Autodesk Inventor part; units mm, degrees
(part 5 of 6)
  arc A594 (139.7365, 123.5324) -> (139.7669, 123.0449) centre (147.3204, 123.76) ccw projected
  arc A595 (140.0993, 123.6997) -> (139.7365, 123.5324) centre (148.5, 105) ccw projected
  arc A596 (140.4503, 123.36) -> (140.0993, 123.6997) centre (135.0009, 118.0806) ccw projected
  arc A597 (140.7158, 123.0684) -> (140.4503, 123.36) centre (135.8481, 118.9014) ccw projected
  arc A598 (140.9107, 122.8267) -> (140.7158, 123.0684) centre (136.7109, 119.64) ccw projected
  arc A599 (141.2611, 122.9719) -> (140.9107, 122.8267) centre (148.5, 105) ccw projected
  arc A600 (141.228, 123.2805) -> (141.2611, 122.9719) centre (146.4841, 123.6882) ccw projected
  arc A601 (141.2096, 123.6745) -> (141.228, 123.2805) centre (147.6165, 123.776) ccw projected
  arc A602 (141.2175, 124.1629) -> (141.2096, 123.6745) centre (148.7959, 123.7947) ccw projected
  arc A603 (141.5923, 124.3011) -> (141.2175, 124.1629) centre (148.5, 105) ccw projected
  arc A604 (141.9156, 123.9349) -> (141.5923, 124.3011) centre (136.0688, 119.0994) ccw projected
  arc A605 (142.1575, 123.6234) -> (141.9156, 123.9349) centre (136.9778, 119.8512) ccw projected
  arc A606 (142.3327, 123.3672) -> (142.1575, 123.6234) centre (137.8959, 120.5199) ccw projected
  arc A607 (142.6934, 123.4844) -> (142.3327, 123.3672) centre (148.5, 105) ccw projected
  arc A608 (142.6846, 123.7947) -> (142.6934, 123.4844) centre (147.9566, 123.7888) ccw projected
  arc A609 (142.6972, 124.1889) -> (142.6846, 123.7947) centre (149.0924, 123.7875) ccw projected
  arc A610 (142.7435, 124.6752) -> (142.6972, 124.1889) centre (150.2696, 123.7136) ccw projected
  arc A611 (143.128, 124.7836) -> (142.7435, 124.6752) centre (148.5, 105) ccw projected
  arc A612 (143.4215, 124.3932) -> (143.128, 124.7836) centre (137.2133, 120.0313) ccw projected
  arc A613 (143.6382, 124.0636) -> (143.4215, 124.3932) centre (138.1785, 120.7095) ccw projected
  arc A614 (143.7928, 123.7945) -> (143.6382, 124.0636) centre (139.1463, 121.304) ccw projected
  arc A615 (144.1616, 123.883) -> (143.7928, 123.7945) centre (148.5, 105) ccw projected
  arc A616 (144.1772, 124.193) -> (144.1616, 123.883) centre (149.4324, 123.7735) ccw projected
  arc A617 (144.2207, 124.585) -> (144.1772, 124.193) centre (150.5646, 123.6831) ccw projected
  arc A618 (144.3049, 125.0662) -> (144.2207, 124.585) centre (151.7324, 123.517) ccw projected
  arc A619 (144.6967, 125.1441) -> (144.3049, 125.0662) centre (148.5, 105) ccw projected
  arc A620 (144.9587, 124.7318) -> (144.6967, 125.1441) centre (138.4274, 120.8705) ccw projected
  arc A621 (145.1489, 124.3863) -> (144.9587, 124.7318) centre (139.4429, 121.4708) ccw projected
  arc A622 (145.2819, 124.1059) -> (145.1489, 124.3863) centre (140.4543, 121.9876) ccw projected
  arc A623 (145.6565, 124.1652) -> (145.2819, 124.1059) centre (148.5, 105) ccw projected
  arc A624 (145.6964, 124.473) -> (145.6565, 124.1652) centre (150.9025, 123.6425) ccw projected
  arc A625 (145.7705, 124.8604) -> (145.6964, 124.473) centre (152.0241, 123.4635) ccw projected
  arc A626 (145.8922, 125.3335) -> (145.7705, 124.8604) centre (153.1753, 123.2064) ccw projected
  arc A627 (146.2889, 125.3804) -> (145.8922, 125.3335) centre (148.5, 105) ccw projected
  arc A628 (146.5178, 124.9489) -> (146.2889, 125.3804) centre (139.7037, 121.6119) ccw projected
  arc A629 (146.6803, 124.5895) -> (146.5178, 124.9489) centre (140.7631, 122.1307) ccw projected
  arc A630 (146.7909, 124.2995) -> (146.6803, 124.5895) centre (141.8119, 122.5665) ccw projected
  arc A631 (147.169, 124.3292) -> (146.7909, 124.2995) centre (148.5, 105) ccw projected
  arc A632 (147.2329, 124.633) -> (147.169, 124.3292) centre (152.3577, 123.3965) ccw projected
  arc A633 (147.3371, 125.0133) -> (147.2329, 124.633) centre (153.4618, 123.1301) ccw projected
  arc A634 (147.4956, 125.4754) -> (147.3371, 125.0133) centre (154.5894, 122.7834) ccw projected
  arc A635 (147.8948, 125.4911) -> (147.4956, 125.4754) centre (148.5, 105) ccw projected
  arc A636 (148.0891, 125.0429) -> (147.8948, 125.4911) centre (141.0342, 122.2508) ccw projected
  arc A637 (148.2229, 124.6719) -> (148.0891, 125.0429) centre (142.131, 122.6849) ccw projected
  arc A638 (148.3104, 124.3741) -> (148.2229, 124.6719) centre (143.2108, 123.0371) ccw projected
  arc A639 (148.6896, 124.3741) -> (148.3104, 124.3741) centre (148.5, 105) ccw projected
  arc A640 (148.7771, 124.6719) -> (148.6896, 124.3741) centre (153.7892, 123.0371) ccw projected
  circle A641 centre (148.5, 105) radius 6
  circle A642 centre (148.5, 105) radius 18.25
  point P0 (0, 0)
  dimension "d15" = 12
  dimension "d16" = 36.5
  constraints: 2 centre point, 2 coincident
  measures "d15" diameter of A641
  measures "d16" diameter of A642
extrude "押し出し4" cut sketch "スケッチ4" against normal blind 0.75 contours A642
fillet "フィレット1" radius 0.5 20 edges at (145.1332, 103.3479, -2.5) (144.8051, 104.3575, -2.5) (144.8051, 105.6424, -2.5) (145.1331, 106.652, -2.5) (145.8883, 107.6915, -2.5) (146.7471, 108.3155, -2.5) (147.9691, 108.7126, -2.5) (149.0314, 108.7125, -2.5) (150.2528, 108.3155, -2.5) (151.1126, 107.6906, -2.5) (151.8668, 106.6521, -2.5) (152.1951, 105.6411, -2.5) (152.1949, 104.3576, -2.5) (151.8663, 103.3467, -2.5) (151.1117, 102.3085, -2.5) (150.2516, 101.6838, -2.5) (149.0308, 101.2874, -2.5) (147.9686, 101.2875, -2.5) (146.7478, 101.6841, -2.5) (145.8884, 102.3084, -2.5)
sketch "スケッチ5" plane through (148.5, 105, 0.75) normal (0, 0, -1) x (-1, 0, 0)
  circle A0 centre (0, 0) radius 6 projected
  circle A1 centre (0, 0) radius 18.25 projected
  circle A2 centre (0, 0) radius 2 projected
  arc A3 (-0.2771, 19.6719) -> (-0.4109, 20.0429) centre (-6.369, 17.6849) ccw projected
  arc A4 (-0.1896, 19.3741) -> (-0.2771, 19.6719) centre (-5.2892, 18.0371) ccw projected
  arc A5 (0.1896, 19.3741) -> (-0.1896, 19.3741) centre (0, 0) ccw projected
  arc A6 (0.2771, 19.6719) -> (0.1896, 19.3741) centre (5.2892, 18.0371) ccw projected
  arc A7 (0.4109, 20.0429) -> (0.2771, 19.6719) centre (6.369, 17.6849) ccw projected
  arc A8 (0.6052, 20.4911) -> (0.4109, 20.0429) centre (7.4658, 17.2508) ccw projected
  arc A9 (1.0044, 20.4754) -> (0.6052, 20.4911) centre (0, 0) ccw projected
  arc A10 (1.1629, 20.0133) -> (1.0044, 20.4754) centre (-6.0894, 17.7834) ccw projected
  arc A11 (1.2671, 19.633) -> (1.1629, 20.0133) centre (-4.9618, 18.1301) ccw projected
  arc A12 (1.331, 19.3292) -> (1.2671, 19.633) centre (-3.8577, 18.3965) ccw projected
  arc A13 (1.7091, 19.2995) -> (1.331, 19.3292) centre (0, 0) ccw projected
  arc A14 (1.8197, 19.5895) -> (1.7091, 19.2995) centre (6.6881, 17.5665) ccw projected
  arc A15 (1.9822, 19.9489) -> (1.8197, 19.5895) centre (7.7369, 17.1307) ccw projected
  arc A16 (2.2111, 20.3804) -> (1.9822, 19.9489) centre (8.7963, 16.6119) ccw projected
  arc A17 (2.6078, 20.3335) -> (2.2111, 20.3804) centre (0, 0) ccw projected
  arc A18 (2.7295, 19.8604) -> (2.6078, 20.3335) centre (-4.6753, 18.2064) ccw projected
  arc A19 (2.8036, 19.473) -> (2.7295, 19.8604) centre (-3.5241, 18.4635) ccw projected
  arc A20 (2.8435, 19.1652) -> (2.8036, 19.473) centre (-2.4025, 18.6425) ccw projected
  arc A21 (3.2181, 19.1059) -> (2.8435, 19.1652) centre (0, 0) ccw projected
  arc A22 (3.3511, 19.3863) -> (3.2181, 19.1059) centre (8.0457, 16.9876) ccw projected
  arc A23 (3.5413, 19.7318) -> (3.3511, 19.3863) centre (9.0571, 16.4708) ccw projected
  arc A24 (3.8033, 20.1441) -> (3.5413, 19.7318) centre (10.0726, 15.8705) ccw projected
  arc A25 (4.1951, 20.0662) -> (3.8033, 20.1441) centre (0, 0) ccw projected
  arc A26 (4.2793, 19.585) -> (4.1951, 20.0662) centre (-3.2324, 18.517) ccw projected
  arc A27 (4.3228, 19.193) -> (4.2793, 19.585) centre (-2.0646, 18.6831) ccw projected
  arc A28 (4.3384, 18.883) -> (4.3228, 19.193) centre (-0.9324, 18.7735) ccw projected
  arc A29 (4.7072, 18.7945) -> (4.3384, 18.883) centre (0, 0) ccw projected
  arc A30 (4.8618, 19.0636) -> (4.7072, 18.7945) centre (9.3537, 16.304) ccw projected
  arc A31 (5.0785, 19.3932) -> (4.8618, 19.0636) centre (10.3215, 15.7095) ccw projected
  arc A32 (5.372, 19.7836) -> (5.0785, 19.3932) centre (11.2867, 15.0313) ccw projected
  arc A33 (5.7565, 19.6752) -> (5.372, 19.7836) centre (0, 0) ccw projected
  arc A34 (5.8028, 19.1889) -> (5.7565, 19.6752) centre (-1.7696, 18.7136) ccw projected
  arc A35 (5.8154, 18.7947) -> (5.8028, 19.1889) centre (-0.5924, 18.7875) ccw projected
  arc A36 (5.8066, 18.4844) -> (5.8154, 18.7947) centre (0.5434, 18.7888) ccw projected
  arc A37 (6.1673, 18.3672) -> (5.8066, 18.4844) centre (0, 0) ccw projected
  arc A38 (6.3425, 18.6234) -> (6.1673, 18.3672) centre (10.6041, 15.5199) ccw projected
  arc A39 (6.5844, 18.9349) -> (6.3425, 18.6234) centre (11.5222, 14.8512) ccw projected
  arc A40 (6.9077, 19.3011) -> (6.5844, 18.9349) centre (12.4312, 14.0994) ccw projected
  arc A41 (7.2825, 19.1629) -> (6.9077, 19.3011) centre (0, 0) ccw projected
  arc A42 (7.2904, 18.6745) -> (7.2825, 19.1629) centre (-0.2959, 18.7947) ccw projected
  arc A43 (7.272, 18.2805) -> (7.2904, 18.6745) centre (0.8835, 18.776) ccw projected
  arc A44 (7.2389, 17.9719) -> (7.272, 18.2805) centre (2.0159, 18.6882) ccw projected
  arc A45 (7.5893, 17.8267) -> (7.2389, 17.9719) centre (0, 0) ccw projected
  arc A46 (7.7842, 18.0684) -> (7.5893, 17.8267) centre (11.7891, 14.64) ccw projected
  arc A47 (8.0497, 18.36) -> (7.7842, 18.0684) centre (12.6519, 13.9014) ccw projected
  arc A48 (8.4007, 18.6997) -> (8.0497, 18.36) centre (13.4991, 13.0806) ccw projected
  arc A49 (8.7635, 18.5324) -> (8.4007, 18.6997) centre (0, 0) ccw projected
  arc A50 (8.7331, 18.0449) -> (8.7635, 18.5324) centre (1.1796, 18.76) ccw projected
  arc A51 (8.6839, 17.6536) -> (8.7331, 18.0449) centre (2.3539, 18.6488) ccw projected
  arc A52 (8.6267, 17.3485) -> (8.6839, 17.6536) centre (3.476, 18.4724) ccw projected
  arc A53 (8.9646, 17.1763) -> (8.6267, 17.3485) centre (0, 0) ccw projected
  arc A54 (9.1778, 17.4019) -> (8.9646, 17.1763) centre (12.9014, 13.6699) ccw projected
  arc A55 (9.4654, 17.6718) -> (9.1778, 17.4019) centre (13.7036, 12.8659) ccw projected
  arc A56 (9.842, 17.9829) -> (9.4654, 17.6718) centre (14.4838, 11.9812) ccw projected
  arc A57 (10.1905, 17.7877) -> (9.842, 17.9829) centre (0, 0) ccw projected
  arc A58 (10.122, 17.3041) -> (10.1905, 17.7877) centre (2.6478, 18.6096) ccw projected
  arc A59 (10.0422, 16.9178) -> (10.122, 17.3041) centre (3.8099, 18.4067) ccw projected
  arc A60 (9.9612, 16.6182) -> (10.0422, 16.9178) centre (4.9146, 18.1428) ccw projected
  arc A61 (10.2846, 16.42) -> (9.9612, 16.6182) centre (0, 0) ccw projected
  arc A62 (10.5148, 16.6282) -> (10.2846, 16.42) centre (13.9341, 12.6156) ccw projected
  arc A63 (10.8227, 16.8747) -> (10.5148, 16.6282) centre (14.6708, 11.7511) ccw projected
  arc A64 (11.2226, 17.1553) -> (10.8227, 16.8747) centre (15.3792, 10.8078) ccw projected
  arc A65 (11.5547, 16.9334) -> (11.2226, 17.1553) centre (0, 0) ccw projected
  arc A66 (11.4485, 16.4566) -> (11.5547, 16.9334) centre (4.0998, 18.3445) ccw projected
  arc A67 (11.3386, 16.0778) -> (11.4485, 16.4566) centre (5.2423, 18.051) ccw projected
  arc A68 (11.2344, 15.7854) -> (11.3386, 16.0778) centre (6.3229, 17.7012) ccw projected
  arc A69 (11.5412, 15.5625) -> (11.2344, 15.7854) centre (0, 0) ccw projected
  arc A70 (11.7871, 15.752) -> (11.5412, 15.5625) centre (14.881, 11.4834) ccw projected
  arc A71 (12.1134, 15.9735) -> (11.7871, 15.752) centre (15.5476, 10.5638) ccw projected
  arc A72 (12.534, 16.2219) -> (12.1134, 15.9735) centre (16.1798, 9.5679) ccw projected
  arc A73 (12.8477, 15.9746) -> (12.534, 16.2219) centre (0, 0) ccw projected
  arc A74 (12.7043, 15.5076) -> (12.8477, 15.9746) centre (5.5264, 17.9663) ccw projected
  arc A75 (12.5651, 15.1386) -> (12.7043, 15.5076) centre (6.6424, 17.5841) ccw projected
  arc A76 (12.4383, 14.8553) -> (12.5651, 15.1386) centre (7.6922, 17.1506) ccw projected
  arc A77 (12.7266, 14.609) -> (12.4383, 14.8553) centre (0, 0) ccw projected
  arc A78 (12.9866, 14.7786) -> (12.7266, 14.609) centre (15.7361, 10.2805) ccw projected
  arc A79 (13.3293, 14.9739) -> (12.9866, 14.7786) centre (16.3285, 9.3114) ccw projected
  arc A80 (13.7681, 15.1885) -> (13.3293, 14.9739) centre (16.8806, 8.2689) ccw projected
  arc A81 (14.0614, 14.9173) -> (13.7681, 15.1885) centre (0, 0) ccw projected
  arc A82 (13.8819, 14.463) -> (14.0614, 14.9173) centre (6.919, 17.4773) ccw projected
  arc A83 (13.7141, 14.1061) -> (13.8819, 14.463) centre (8.0015, 17.0087) ccw projected
  arc A84 (13.5655, 13.8336) -> (13.7141, 14.1061) centre (9.0141, 16.4942) ccw projected
  arc A85 (13.8336, 13.5655) -> (13.5655, 13.8336) centre (0, 0) ccw projected
  arc A86 (14.1061, 13.7141) -> (13.8336, 13.5655) centre (16.4942, 9.0141) ccw projected
  arc A87 (14.463, 13.8819) -> (14.1061, 13.7141) centre (17.0087, 8.0015) ccw projected
  arc A88 (14.9173, 14.0614) -> (14.463, 13.8819) centre (17.4773, 6.919) ccw projected
  arc A89 (15.1885, 13.7681) -> (14.9173, 14.0614) centre (0, 0) ccw projected
  arc A90 (14.9739, 13.3293) -> (15.1885, 13.7681) centre (8.2689, 16.8806) ccw projected
  arc A91 (14.7786, 12.9866) -> (14.9739, 13.3293) centre (9.3114, 16.3285) ccw projected
  arc A92 (14.609, 12.7266) -> (14.7786, 12.9866) centre (10.2805, 15.7361) ccw projected
  arc A93 (14.8553, 12.4383) -> (14.609, 12.7266) centre (0, 0) ccw projected
  arc A94 (15.1386, 12.5651) -> (14.8553, 12.4383) centre (17.1506, 7.6922) ccw projected
  arc A95 (15.5076, 12.7043) -> (15.1386, 12.5651) centre (17.5841, 6.6424) ccw projected
  arc A96 (15.9746, 12.8477) -> (15.5076, 12.7043) centre (17.9663, 5.5264) ccw projected
  arc A97 (16.2219, 12.534) -> (15.9746, 12.8477) centre (0, 0) ccw projected
  arc A98 (15.9735, 12.1134) -> (16.2219, 12.534) centre (9.5679, 16.1798) ccw projected
  arc A99 (15.752, 11.7871) -> (15.9735, 12.1134) centre (10.5638, 15.5476) ccw projected
  arc A100 (15.5625, 11.5412) -> (15.752, 11.7871) centre (11.4834, 14.881) ccw projected
  arc A101 (15.7854, 11.2344) -> (15.5625, 11.5412) centre (0, 0) ccw projected
  arc A102 (16.0778, 11.3386) -> (15.7854, 11.2344) centre (17.7012, 6.3229) ccw projected
  arc A103 (16.4566, 11.4485) -> (16.0778, 11.3386) centre (18.051, 5.2423) ccw projected
  arc A104 (16.9334, 11.5547) -> (16.4566, 11.4485) centre (18.3445, 4.0998) ccw projected
  arc A105 (17.1553, 11.2226) -> (16.9334, 11.5547) centre (0, 0) ccw projected
  arc A106 (16.8747, 10.8227) -> (17.1553, 11.2226) centre (10.8078, 15.3792) ccw projected
  arc A107 (16.6282, 10.5148) -> (16.8747, 10.8227) centre (11.7511, 14.6708) ccw projected
  arc A108 (16.42, 10.2846) -> (16.6282, 10.5148) centre (12.6156, 13.9341) ccw projected
  arc A109 (16.6182, 9.9612) -> (16.42, 10.2846) centre (0, 0) ccw projected
  arc A110 (16.9178, 10.0422) -> (16.6182, 9.9612) centre (18.1428, 4.9146) ccw projected
  arc A111 (17.3041, 10.122) -> (16.9178, 10.0422) centre (18.4067, 3.8099) ccw projected
  arc A112 (17.7877, 10.1905) -> (17.3041, 10.122) centre (18.6096, 2.6478) ccw projected
  arc A113 (17.9829, 9.842) -> (17.7877, 10.1905) centre (0, 0) ccw projected
  arc A114 (17.6718, 9.4654) -> (17.9829, 9.842) centre (11.9812, 14.4838) ccw projected
  arc A115 (17.4019, 9.1778) -> (17.6718, 9.4654) centre (12.8659, 13.7036) ccw projected
  arc A116 (17.1763, 8.9646) -> (17.4019, 9.1778) centre (13.6699, 12.9014) ccw projected
  arc A117 (17.3485, 8.6267) -> (17.1763, 8.9646) centre (0, 0) ccw projected
  arc A118 (17.6536, 8.6839) -> (17.3485, 8.6267) centre (18.4724, 3.476) ccw projected
  arc A119 (18.0449, 8.7331) -> (17.6536, 8.6839) centre (18.6488, 2.3539) ccw projected
  arc A120 (18.5324, 8.7635) -> (18.0449, 8.7331) centre (18.76, 1.1796) ccw projected
  arc A121 (18.6997, 8.4007) -> (18.5324, 8.7635) centre (0, 0) ccw projected
  arc A122 (18.36, 8.0497) -> (18.6997, 8.4007) centre (13.0806, 13.4991) ccw projected
  arc A123 (18.0684, 7.7842) -> (18.36, 8.0497) centre (13.9014, 12.6519) ccw projected
  arc A124 (17.8267, 7.5893) -> (18.0684, 7.7842) centre (14.64, 11.7891) ccw projected
  arc A125 (17.9719, 7.2389) -> (17.8267, 7.5893) centre (0, 0) ccw projected
  arc A126 (18.2805, 7.272) -> (17.9719, 7.2389) centre (18.6882, 2.0159) ccw projected
  arc A127 (18.6745, 7.2904) -> (18.2805, 7.272) centre (18.776, 0.8835) ccw projected
  arc A128 (19.1629, 7.2825) -> (18.6745, 7.2904) centre (18.7947, -0.2959) ccw projected
  arc A129 (19.3011, 6.9077) -> (19.1629, 7.2825) centre (0, 0) ccw projected
  arc A130 (18.9349, 6.5844) -> (19.3011, 6.9077) centre (14.0994, 12.4312) ccw projected
  arc A131 (18.6234, 6.3425) -> (18.9349, 6.5844) centre (14.8512, 11.5222) ccw projected
  arc A132 (18.3672, 6.1673) -> (18.6234, 6.3425) centre (15.5199, 10.6041) ccw projected
  arc A133 (18.4844, 5.8066) -> (18.3672, 6.1673) centre (0, 0) ccw projected
  arc A134 (18.7947, 5.8154) -> (18.4844, 5.8066) centre (18.7888, 0.5434) ccw projected
  arc A135 (19.1889, 5.8028) -> (18.7947, 5.8154) centre (18.7875, -0.5924) ccw projected
  arc A136 (19.6752, 5.7565) -> (19.1889, 5.8028) centre (18.7136, -1.7696) ccw projected
  arc A137 (19.7836, 5.372) -> (19.6752, 5.7565) centre (0, 0) ccw projected
  arc A138 (19.3932, 5.0785) -> (19.7836, 5.372) centre (15.0313, 11.2867) ccw projected
  arc A139 (19.0636, 4.8618) -> (19.3932, 5.0785) centre (15.7095, 10.3215) ccw projected
  arc A140 (18.7945, 4.7072) -> (19.0636, 4.8618) centre (16.304, 9.3537) ccw projected
  arc A141 (18.883, 4.3384) -> (18.7945, 4.7072) centre (0, 0) ccw projected
  arc A142 (19.193, 4.3228) -> (18.883, 4.3384) centre (18.7735, -0.9324) ccw projected
  arc A143 (19.585, 4.2793) -> (19.193, 4.3228) centre (18.6831, -2.0646) ccw projected
  arc A144 (20.0662, 4.1951) -> (19.585, 4.2793) centre (18.517, -3.2324) ccw projected
  arc A145 (20.1441, 3.8033) -> (20.0662, 4.1951) centre (0, 0) ccw projected
  arc A146 (19.7318, 3.5413) -> (20.1441, 3.8033) centre (15.8705, 10.0726) ccw projected
  arc A147 (19.3863, 3.3511) -> (19.7318, 3.5413) centre (16.4708, 9.0571) ccw projected
  arc A148 (19.1059, 3.2181) -> (19.3863, 3.3511) centre (16.9876, 8.0457) ccw projected
  arc A149 (19.1652, 2.8435) -> (19.1059, 3.2181) centre (0, 0) ccw projected
  arc A150 (19.473, 2.8036) -> (19.1652, 2.8435) centre (18.6425, -2.4025) ccw projected
  arc A151 (19.8604, 2.7295) -> (19.473, 2.8036) centre (18.4635, -3.5241) ccw projected
  arc A152 (20.3335, 2.6078) -> (19.8604, 2.7295) centre (18.2064, -4.6753) ccw projected
  arc A153 (20.3804, 2.2111) -> (20.3335, 2.6078) centre (0, 0) ccw projected
  arc A154 (19.9489, 1.9822) -> (20.3804, 2.2111) centre (16.6119, 8.7963) ccw projected
  arc A155 (19.5895, 1.8197) -> (19.9489, 1.9822) centre (17.1307, 7.7369) ccw projected
  arc A156 (19.2995, 1.7091) -> (19.5895, 1.8197) centre (17.5665, 6.6881) ccw projected
  arc A157 (19.3292, 1.331) -> (19.2995, 1.7091) centre (0, 0) ccw projected
  arc A158 (19.633, 1.2671) -> (19.3292, 1.331) centre (18.3965, -3.8577) ccw projected
  arc A159 (20.0133, 1.1629) -> (19.633, 1.2671) centre (18.1301, -4.9618) ccw projected
  arc A160 (20.4754, 1.0044) -> (20.0133, 1.1629) centre (17.7834, -6.0894) ccw projected
  arc A161 (20.4911, 0.6052) -> (20.4754, 1.0044) centre (0, 0) ccw projected
  arc A162 (20.0429, 0.4109) -> (20.4911, 0.6052) centre (17.2508, 7.4658) ccw projected
  arc A163 (19.6719, 0.2771) -> (20.0429, 0.4109) centre (17.6849, 6.369) ccw projected
  arc A164 (19.3741, 0.1896) -> (19.6719, 0.2771) centre (18.0371, 5.2892) ccw projected
  arc A165 (19.3741, -0.1896) -> (19.3741, 0.1896) centre (0, 0) ccw projected
  arc A166 (19.6719, -0.2771) -> (19.3741, -0.1896) centre (18.0371, -5.2892) ccw projected
  arc A167 (20.0429, -0.4109) -> (19.6719, -0.2771) centre (17.6849, -6.369) ccw projected
  arc A168 (20.4911, -0.6052) -> (20.0429, -0.4109) centre (17.2508, -7.4658) ccw projected
  arc A169 (20.4754, -1.0044) -> (20.4911, -0.6052) centre (0, 0) ccw projected
  arc A170 (20.0133, -1.1629) -> (20.4754, -1.0044) centre (17.7834, 6.0894) ccw projected
  arc A171 (19.633, -1.2671) -> (20.0133, -1.1629) centre (18.1301, 4.9618) ccw projected
  arc A172 (19.3292, -1.331) -> (19.633, -1.2671) centre (18.3965, 3.8577) ccw projected
  arc A173 (19.2995, -1.7091) -> (19.3292, -1.331) centre (0, 0) ccw projected
  arc A174 (19.5895, -1.8197) -> (19.2995, -1.7091) centre (17.5665, -6.6881) ccw projected
  arc A175 (19.9489, -1.9822) -> (19.5895, -1.8197) centre (17.1307, -7.7369) ccw projected
  arc A176 (20.3804, -2.2111) -> (19.9489, -1.9822) centre (16.6119, -8.7963) ccw projected
  arc A177 (20.3335, -2.6078) -> (20.3804, -2.2111) centre (0, 0) ccw projected
  arc A178 (19.8604, -2.7295) -> (20.3335, -2.6078) centre (18.2064, 4.6753) ccw projected
  arc A179 (19.473, -2.8036) -> (19.8604, -2.7295) centre (18.4635, 3.5241) ccw projected
  arc A180 (19.1652, -2.8435) -> (19.473, -2.8036) centre (18.6425, 2.4025) ccw projected
  arc A181 (19.1059, -3.2181) -> (19.1652, -2.8435) centre (0, 0) ccw projected
  arc A182 (19.3863, -3.3511) -> (19.1059, -3.2181) centre (16.9876, -8.0457) ccw projected
  arc A183 (19.7318, -3.5413) -> (19.3863, -3.3511) centre (16.4708, -9.0571) ccw projected
  arc A184 (20.1441, -3.8033) -> (19.7318, -3.5413) centre (15.8705, -10.0726) ccw projected
  arc A185 (20.0662, -4.1951) -> (20.1441, -3.8033) centre (0, 0) ccw projected
  arc A186 (19.585, -4.2793) -> (20.0662, -4.1951) centre (18.517, 3.2324) ccw projected
  arc A187 (19.193, -4.3228) -> (19.585, -4.2793) centre (18.6831, 2.0646) ccw projected
  arc A188 (18.883, -4.3384) -> (19.193, -4.3228) centre (18.7735, 0.9324) ccw projected
  arc A189 (18.7945, -4.7072) -> (18.883, -4.3384) centre (0, 0) ccw projected
  arc A190 (19.0636, -4.8618) -> (18.7945, -4.7072) centre (16.304, -9.3537) ccw projected
  arc A191 (19.3932, -5.0785) -> (19.0636, -4.8618) centre (15.7095, -10.3215) ccw projected
  arc A192 (19.7836, -5.372) -> (19.3932, -5.0785) centre (15.0313, -11.2867) ccw projected
  arc A193 (19.6752, -5.7565) -> (19.7836, -5.372) centre (0, 0) ccw projected
  arc A194 (19.1889, -5.8028) -> (19.6752, -5.7565) centre (18.7136, 1.7696) ccw projected
  arc A195 (18.7947, -5.8154) -> (19.1889, -5.8028) centre (18.7875, 0.5924) ccw projected
  arc A196 (18.4844, -5.8066) -> (18.7947, -5.8154) centre (18.7888, -0.5434) ccw projected
  arc A197 (18.3672, -6.1673) -> (18.4844, -5.8066) centre (0, 0) ccw projected
  arc A198 (18.6234, -6.3425) -> (18.3672, -6.1673) centre (15.5199, -10.6041) ccw projected
  arc A199 (18.9349, -6.5844) -> (18.6234, -6.3425) centre (14.8512, -11.5222) ccw projected
  arc A200 (19.3011, -6.9077) -> (18.9349, -6.5844) centre (14.0994, -12.4312) ccw projected
  arc A201 (19.1629, -7.2825) -> (19.3011, -6.9077) centre (0, 0) ccw projected
  arc A202 (18.6745, -7.2904) -> (19.1629, -7.2825) centre (18.7947, 0.2959) ccw projected
  arc A203 (18.2805, -7.272) -> (18.6745, -7.2904) centre (18.776, -0.8835) ccw projected
  arc A204 (17.9719, -7.2389) -> (18.2805, -7.272) centre (18.6882, -2.0159) ccw projected
  arc A205 (17.8267, -7.5893) -> (17.9719, -7.2389) centre (0, 0) ccw projected
  arc A206 (18.0684, -7.7842) -> (17.8267, -7.5893) centre (14.64, -11.7891) ccw projected
  arc A207 (18.36, -8.0497) -> (18.0684, -7.7842) centre (13.9014, -12.6519) ccw projected
  arc A208 (18.6997, -8.4007) -> (18.36, -8.0497) centre (13.0806, -13.4991) ccw projected
  arc A209 (18.5324, -8.7635) -> (18.6997, -8.4007) centre (0, 0) ccw projected
  arc A210 (18.0449, -8.7331) -> (18.5324, -8.7635) centre (18.76, -1.1796) ccw projected
  arc A211 (17.6536, -8.6839) -> (18.0449, -8.7331) centre (18.6488, -2.3539) ccw projected
  arc A212 (17.3485, -8.6267) -> (17.6536, -8.6839) centre (18.4724, -3.476) ccw projected
  arc A213 (17.1763, -8.9646) -> (17.3485, -8.6267) centre (0, 0) ccw projected
  arc A214 (17.4019, -9.1778) -> (17.1763, -8.9646) centre (13.6699, -12.9014) ccw projected
  arc A215 (17.6718, -9.4654) -> (17.4019, -9.1778) centre (12.8659, -13.7036) ccw projected
  arc A216 (17.9829, -9.842) -> (17.6718, -9.4654) centre (11.9812, -14.4838) ccw projected
  arc A217 (17.7877, -10.1905) -> (17.9829, -9.842) centre (0, 0) ccw projected
  arc A218 (17.3041, -10.122) -> (17.7877, -10.1905) centre (18.6096, -2.6478) ccw projected
  arc A219 (16.9178, -10.0422) -> (17.3041, -10.122) centre (18.4067, -3.8099) ccw projected
  arc A220 (16.6182, -9.9612) -> (16.9178, -10.0422) centre (18.1428, -4.9146) ccw projected
  arc A221 (16.42, -10.2846) -> (16.6182, -9.9612) centre (0, 0) ccw projected
  arc A222 (16.6282, -10.5148) -> (16.42, -10.2846) centre (12.6156, -13.9341) ccw projected
  arc A223 (16.8747, -10.8227) -> (16.6282, -10.5148) centre (11.7511, -14.6708) ccw projected
  arc A224 (17.1553, -11.2226) -> (16.8747, -10.8227) centre (10.8078, -15.3792) ccw projected
  arc A225 (16.9334, -11.5547) -> (17.1553, -11.2226) centre (0, 0) ccw projected
  arc A226 (16.4566, -11.4485) -> (16.9334, -11.5547) centre (18.3445, -4.0998) ccw projected
  arc A227 (16.0778, -11.3386) -> (16.4566, -11.4485) centre (18.051, -5.2423) ccw projected
  arc A228 (15.7854, -11.2344) -> (16.0778, -11.3386) centre (17.7012, -6.3229) ccw projected
  arc A229 (15.5625, -11.5412) -> (15.7854, -11.2344) centre (0, 0) ccw projected
  arc A230 (15.752, -11.7871) -> (15.5625, -11.5412) centre (11.4834, -14.881) ccw projected
  arc A231 (15.9735, -12.1134) -> (15.752, -11.7871) centre (10.5638, -15.5476) ccw projected
  arc A232 (16.2219, -12.534) -> (15.9735, -12.1134) centre (9.5679, -16.1798) ccw projected
  arc A233 (15.9746, -12.8477) -> (16.2219, -12.534) centre (0, 0) ccw projected
  arc A234 (15.5076, -12.7043) -> (15.9746, -12.8477) centre (17.9663, -5.5264) ccw projected
  arc A235 (15.1386, -12.5651) -> (15.5076, -12.7043) centre (17.5841, -6.6424) ccw projected
  arc A236 (14.8553, -12.4383) -> (15.1386, -12.5651) centre (17.1506, -7.6922) ccw projected
  arc A237 (14.609, -12.7266) -> (14.8553, -12.4383) centre (0, 0) ccw projected
  arc A238 (14.7786, -12.9866) -> (14.609, -12.7266) centre (10.2805, -15.7361) ccw projected
  arc A239 (14.9739, -13.3293) -> (14.7786, -12.9866) centre (9.3114, -16.3285) ccw projected
  arc A240 (15.1885, -13.7681) -> (14.9739, -13.3293) centre (8.2689, -16.8806) ccw projected
  arc A241 (14.9173, -14.0614) -> (15.1885, -13.7681) centre (0, 0) ccw projected
  arc A242 (14.463, -13.8819) -> (14.9173, -14.0614) centre (17.4773, -6.919) ccw projected
  arc A243 (14.1061, -13.7141) -> (14.463, -13.8819) centre (17.0087, -8.0015) ccw projected
  arc A244 (13.8336, -13.5655) -> (14.1061, -13.7141) centre (16.4942, -9.0141) ccw projected
  arc A245 (13.5655, -13.8336) -> (13.8336, -13.5655) centre (0, 0) ccw projected
  arc A246 (13.7141, -14.1061) -> (13.5655, -13.8336) centre (9.0141, -16.4942) ccw projected
  arc A247 (13.8819, -14.463) -> (13.7141, -14.1061) centre (8.0015, -17.0087) ccw projected
  arc A248 (14.0614, -14.9173) -> (13.8819, -14.463) centre (6.919, -17.4773) ccw projected
  arc A249 (13.7681, -15.1885) -> (14.0614, -14.9173) centre (0, 0) ccw projected
  arc A250 (13.3293, -14.9739) -> (13.7681, -15.1885) centre (16.8806, -8.2689) ccw projected
  arc A251 (12.9866, -14.7786) -> (13.3293, -14.9739) centre (16.3285, -9.3114) ccw projected
  arc A252 (12.7266, -14.609) -> (12.9866, -14.7786) centre (15.7361, -10.2805) ccw projected
  arc A253 (12.4383, -14.8553) -> (12.7266, -14.609) centre (0, 0) ccw projected
  arc A254 (12.5651, -15.1386) -> (12.4383, -14.8553) centre (7.6922, -17.1506) ccw projected
  arc A255 (12.7043, -15.5076) -> (12.5651, -15.1386) centre (6.6424, -17.5841) ccw projected
  arc A256 (12.8477, -15.9746) -> (12.7043, -15.5076) centre (5.5264, -17.9663) ccw projected
  arc A257 (12.534, -16.2219) -> (12.8477, -15.9746) centre (0, 0) ccw projected
  arc A258 (12.1134, -15.9735) -> (12.534, -16.2219) centre (16.1798, -9.5679) ccw projected
  arc A259 (11.7871, -15.752) -> (12.1134, -15.9735) centre (15.5476, -10.5638) ccw projected
  arc A260 (11.5412, -15.5625) -> (11.7871, -15.752) centre (14.881, -11.4834) ccw projected
  arc A261 (11.2344, -15.7854) -> (11.5412, -15.5625) centre (0, 0) ccw projected
  arc A262 (11.3386, -16.0778) -> (11.2344, -15.7854) centre (6.3229, -17.7012) ccw projected
  arc A263 (11.4485, -16.4566) -> (11.3386, -16.0778) centre (5.2423, -18.051) ccw projected
  arc A264 (11.5547, -16.9334) -> (11.4485, -16.4566) centre (4.0998, -18.3445) ccw projected
  arc A265 (11.2226, -17.1553) -> (11.5547, -16.9334) centre (0, 0) ccw projected
  arc A266 (10.8227, -16.8747) -> (11.2226, -17.1553) centre (15.3792, -10.8078) ccw projected
  arc A267 (10.5148, -16.6282) -> (10.8227, -16.8747) centre (14.6708, -11.7511) ccw projected
  arc A268 (10.2846, -16.42) -> (10.5148, -16.6282) centre (13.9341, -12.6156) ccw projected
  arc A269 (9.9612, -16.6182) -> (10.2846, -16.42) centre (0, 0) ccw projected
  arc A270 (10.0422, -16.9178) -> (9.9612, -16.6182) centre (4.9146, -18.1428) ccw projected
  arc A271 (10.122, -17.3041) -> (10.0422, -16.9178) centre (3.8099, -18.4067) ccw projected
  arc A272 (10.1905, -17.7877) -> (10.122, -17.3041) centre (2.6478, -18.6096) ccw projected
  arc A273 (9.842, -17.9829) -> (10.1905, -17.7877) centre (0, 0) ccw projected
  arc A274 (9.4654, -17.6718) -> (9.842, -17.9829) centre (14.4838, -11.9812) ccw projected
  arc A275 (9.1778, -17.4019) -> (9.4654, -17.6718) centre (13.7036, -12.8659) ccw projected
  arc A276 (8.9646, -17.1763) -> (9.1778, -17.4019) centre (12.9014, -13.6699) ccw projected
  arc A277 (8.6267, -17.3485) -> (8.9646, -17.1763) centre (0, 0) ccw projected
  arc A278 (8.6839, -17.6536) -> (8.6267, -17.3485) centre (3.476, -18.4724) ccw projected
  arc A279 (8.7331, -18.0449) -> (8.6839, -17.6536) centre (2.3539, -18.6488) ccw projected
  arc A280 (8.7635, -18.5324) -> (8.7331, -18.0449) centre (1.1796, -18.76) ccw projected
  arc A281 (8.4007, -18.6997) -> (8.7635, -18.5324) centre (0, 0) ccw projected
  arc A282 (8.0497, -18.36) -> (8.4007, -18.6997) centre (13.4991, -13.0806) ccw projected
  arc A283 (7.7842, -18.0684) -> (8.0497, -18.36) centre (12.6519, -13.9014) ccw projected
  arc A284 (7.5893, -17.8267) -> (7.7842, -18.0684) centre (11.7891, -14.64) ccw projected
  arc A285 (7.2389, -17.9719) -> (7.5893, -17.8267) centre (0, 0) ccw projected
  arc A286 (7.272, -18.2805) -> (7.2389, -17.9719) centre (2.0159, -18.6882) ccw projected
  arc A287 (7.2904, -18.6745) -> (7.272, -18.2805) centre (0.8835, -18.776) ccw projected
  arc A288 (7.2825, -19.1629) -> (7.2904, -18.6745) centre (-0.2959, -18.7947) ccw projected
  arc A289 (6.9077, -19.3011) -> (7.2825, -19.1629) centre (0, 0) ccw projected
  arc A290 (6.5844, -18.9349) -> (6.9077, -19.3011) centre (12.4312, -14.0994) ccw projected
  arc A291 (6.3425, -18.6234) -> (6.5844, -18.9349) centre (11.5222, -14.8512) ccw projected
  arc A292 (6.1673, -18.3672) -> (6.3425, -18.6234) centre (10.6041, -15.5199) ccw projected
  arc A293 (5.8066, -18.4844) -> (6.1673, -18.3672) centre (0, 0) ccw projected
  arc A294 (5.8154, -18.7947) -> (5.8066, -18.4844) centre (0.5434, -18.7888) ccw projected
  arc A295 (5.8028, -19.1889) -> (5.8154, -18.7947) centre (-0.5924, -18.7875) ccw projected
  arc A296 (5.7565, -19.6752) -> (5.8028, -19.1889) centre (-1.7696, -18.7136) ccw projected
  arc A297 (5.372, -19.7836) -> (5.7565, -19.6752) centre (0, 0) ccw projected
  arc A298 (5.0785, -19.3932) -> (5.372, -19.7836) centre (11.2867, -15.0313) ccw projected
  arc A299 (4.8618, -19.0636) -> (5.0785, -19.3932) centre (10.3215, -15.7095) ccw projected
  arc A300 (4.7072, -18.7945) -> (4.8618, -19.0636) centre (9.3537, -16.304) ccw projected
  arc A301 (4.3384, -18.883) -> (4.7072, -18.7945) centre (0, 0) ccw projected
  arc A302 (4.3228, -19.193) -> (4.3384, -18.883) centre (-0.9324, -18.7735) ccw projected
  arc A303 (4.2793, -19.585) -> (4.3228, -19.193) centre (-2.0646, -18.6831) ccw projected
  arc A304 (4.1951, -20.0662) -> (4.2793, -19.585) centre (-3.2324, -18.517) ccw projected
  arc A305 (3.8033, -20.1441) -> (4.1951, -20.0662) centre (0, 0) ccw projected
  arc A306 (3.5413, -19.7318) -> (3.8033, -20.1441) centre (10.0726, -15.8705) ccw projected
  arc A307 (3.3511, -19.3863) -> (3.5413, -19.7318) centre (9.0571, -16.4708) ccw projected
  arc A308 (3.2181, -19.1059) -> (3.3511, -19.3863) centre (8.0457, -16.9876) ccw projected
  arc A309 (2.8435, -19.1652) -> (3.2181, -19.1059) centre (0, 0) ccw projected
  arc A310 (2.8036, -19.473) -> (2.8435, -19.1652) centre (-2.4025, -18.6425) ccw projected
  arc A311 (2.7295, -19.8604) -> (2.8036, -19.473) centre (-3.5241, -18.4635) ccw projected
  arc A312 (2.6078, -20.3335) -> (2.7295, -19.8604) centre (-4.6753, -18.2064) ccw projected
  arc A313 (2.2111, -20.3804) -> (2.6078, -20.3335) centre (0, 0) ccw projected
  arc A314 (1.9822, -19.9489) -> (2.2111, -20.3804) centre (8.7963, -16.6119) ccw projected
  arc A315 (1.8197, -19.5895) -> (1.9822, -19.9489) centre (7.7369, -17.1307) ccw projected
  arc A316 (1.7091, -19.2995) -> (1.8197, -19.5895) centre (6.6881, -17.5665) ccw projected
  arc A317 (1.331, -19.3292) -> (1.7091, -19.2995) centre (0, 0) ccw projected
  arc A318 (1.2671, -19.633) -> (1.331, -19.3292) centre (-3.8577, -18.3965) ccw projected
  arc A319 (1.1629, -20.0133) -> (1.2671, -19.633) centre (-4.9618, -18.1301) ccw projected
  arc A320 (1.0044, -20.4754) -> (1.1629, -20.0133) centre (-6.0894, -17.7834) ccw projected
  arc A321 (0.6052, -20.4911) -> (1.0044, -20.4754) centre (0, 0) ccw projected
  arc A322 (0.4109, -20.0429) -> (0.6052, -20.4911) centre (7.4658, -17.2508) ccw projected
  arc A323 (0.2771, -19.6719) -> (0.4109, -20.0429) centre (6.369, -17.6849) ccw projected
  arc A324 (0.1896, -19.3741) -> (0.2771, -19.6719) centre (5.2892, -18.0371) ccw projected
  arc A325 (-0.1896, -19.3741) -> (0.1896, -19.3741) centre (0, 0) ccw projected
  arc A326 (-0.2771, -19.6719) -> (-0.1896, -19.3741) centre (-5.2892, -18.0371) ccw projected
  arc A327 (-0.4109, -20.0429) -> (-0.2771, -19.6719) centre (-6.369, -17.6849) ccw projected
  arc A328 (-0.6052, -20.4911) -> (-0.4109, -20.0429) centre (-7.4658, -17.2508) ccw projected
  arc A329 (-1.0044, -20.4754) -> (-0.6052, -20.4911) centre (0, 0) ccw projected
  arc A330 (-1.1629, -20.0133) -> (-1.0044, -20.4754) centre (6.0894, -17.7834) ccw projected
  arc A331 (-1.2671, -19.633) -> (-1.1629, -20.0133) centre (4.9618, -18.1301) ccw projected
  arc A332 (-1.331, -19.3292) -> (-1.2671, -19.633) centre (3.8577, -18.3965) ccw projected
  arc A333 (-1.7091, -19.2995) -> (-1.331, -19.3292) centre (0, 0) ccw projected
  arc A334 (-1.8197, -19.5895) -> (-1.7091, -19.2995) centre (-6.6881, -17.5665) ccw projected
  arc A335 (-1.9822, -19.9489) -> (-1.8197, -19.5895) centre (-7.7369, -17.1307) ccw projected
  arc A336 (-2.2111, -20.3804) -> (-1.9822, -19.9489) centre (-8.7963, -16.6119) ccw projected
  arc A337 (-2.6078, -20.3335) -> (-2.2111, -20.3804) centre (0, 0) ccw projected
  arc A338 (-2.7295, -19.8604) -> (-2.6078, -20.3335) centre (4.6753, -18.2064) ccw projected
  arc A339 (-2.8036, -19.473) -> (-2.7295, -19.8604) centre (3.5241, -18.4635) ccw projected
  arc A340 (-2.8435, -19.1652) -> (-2.8036, -19.473) centre (2.4025, -18.6425) ccw projected
  arc A341 (-3.2181, -19.1059) -> (-2.8435, -19.1652) centre (0, 0) ccw projected
  arc A342 (-3.3511, -19.3863) -> (-3.2181, -19.1059) centre (-8.0457, -16.9876) ccw projected
  arc A343 (-3.5413, -19.7318) -> (-3.3511, -19.3863) centre (-9.0571, -16.4708) ccw projected
  arc A344 (-3.8033, -20.1441) -> (-3.5413, -19.7318) centre (-10.0726, -15.8705) ccw projected
  arc A345 (-4.1951, -20.0662) -> (-3.8033, -20.1441) centre (0, 0) ccw projected
  arc A346 (-4.2793, -19.585) -> (-4.1951, -20.0662) centre (3.2324, -18.517) ccw projected
  arc A347 (-4.3228, -19.193) -> (-4.2793, -19.585) centre (2.0646, -18.6831) ccw projected
  arc A348 (-4.3384, -18.883) -> (-4.3228, -19.193) centre (0.9324, -18.7735) ccw projected
  arc A349 (-4.7072, -18.7945) -> (-4.3384, -18.883) centre (0, 0) ccw projected
  arc A350 (-4.8618, -19.0636) -> (-4.7072, -18.7945) centre (-9.3537, -16.304) ccw projected
  arc A351 (-5.0785, -19.3932) -> (-4.8618, -19.0636) centre (-10.3215, -15.7095) ccw projected
  arc A352 (-5.372, -19.7836) -> (-5.0785, -19.3932) centre (-11.2867, -15.0313) ccw projected
  arc A353 (-5.7565, -19.6752) -> (-5.372, -19.7836) centre (0, 0) ccw projected
  arc A354 (-5.8028, -19.1889) -> (-5.7565, -19.6752) centre (1.7696, -18.7136) ccw projected
  arc A355 (-5.8154, -18.7947) -> (-5.8028, -19.1889) centre (0.5924, -18.7875) ccw projected
  arc A356 (-5.8066, -18.4844) -> (-5.8154, -18.7947) centre (-0.5434, -18.7888) ccw projected
  arc A357 (-6.1673, -18.3672) -> (-5.8066, -18.4844) centre (0, 0) ccw projected
  arc A358 (-6.3425, -18.6234) -> (-6.1673, -18.3672) centre (-10.6041, -15.5199) ccw projected
  arc A359 (-6.5844, -18.9349) -> (-6.3425, -18.6234) centre (-11.5222, -14.8512) ccw projected
  arc A360 (-6.9077, -19.3011) -> (-6.5844, -18.9349) centre (-12.4312, -14.0994) ccw projected
  arc A361 (-7.2825, -19.1629) -> (-6.9077, -19.3011) centre (0, 0) ccw projected
  arc A362 (-7.2904, -18.6745) -> (-7.2825, -19.1629) centre (0.2959, -18.7947) ccw projected
  arc A363 (-7.272, -18.2805) -> (-7.2904, -18.6745) centre (-0.8835, -18.776) ccw projected
  arc A364 (-7.2389, -17.9719) -> (-7.272, -18.2805) centre (-2.0159, -18.6882) ccw projected
  arc A365 (-7.5893, -17.8267) -> (-7.2389, -17.9719) centre (0, 0) ccw projected
  arc A366 (-7.7842, -18.0684) -> (-7.5893, -17.8267) centre (-11.7891, -14.64) ccw projected
  arc A367 (-8.0497, -18.36) -> (-7.7842, -18.0684) centre (-12.6519, -13.9014) ccw projected
  arc A368 (-8.4007, -18.6997) -> (-8.0497, -18.36) centre (-13.4991, -13.0806) ccw projected
  arc A369 (-8.7635, -18.5324) -> (-8.4007, -18.6997) centre (0, 0) ccw projected
  arc A370 (-8.7331, -18.0449) -> (-8.7635, -18.5324) centre (-1.1796, -18.76) ccw projected
  arc A371 (-8.6839, -17.6536) -> (-8.7331, -18.0449) centre (-2.3539, -18.6488) ccw projected
  arc A372 (-8.6267, -17.3485) -> (-8.6839, -17.6536) centre (-3.476, -18.4724) ccw projected
  arc A373 (-8.9646, -17.1763) -> (-8.6267, -17.3485) centre (0, 0) ccw projected
  arc A374 (-9.1778, -17.4019) -> (-8.9646, -17.1763) centre (-12.9014, -13.6699) ccw projected
  arc A375 (-9.4654, -17.6718) -> (-9.1778, -17.4019) centre (-13.7036, -12.8659) ccw projected
  arc A376 (-9.842, -17.9829) -> (-9.4654, -17.6718) centre (-14.4838, -11.9812) ccw projected
  arc A377 (-10.1905, -17.7877) -> (-9.842, -17.9829) centre (0, 0) ccw projected
  arc A378 (-10.122, -17.3041) -> (-10.1905, -17.7877) centre (-2.6478, -18.6096) ccw projected
  arc A379 (-10.0422, -16.9178) -> (-10.122, -17.3041) centre (-3.8099, -18.4067) ccw projected
  arc A380 (-9.9612, -16.6182) -> (-10.0422, -16.9178) centre (-4.9146, -18.1428) ccw projected
  arc A381 (-10.2846, -16.42) -> (-9.9612, -16.6182) centre (0, 0) ccw projected
  arc A382 (-10.5148, -16.6282) -> (-10.2846, -16.42) centre (-13.9341, -12.6156) ccw projected
  arc A383 (-10.8227, -16.8747) -> (-10.5148, -16.6282) centre (-14.6708, -11.7511) ccw projected
  arc A384 (-11.2226, -17.1553) -> (-10.8227, -16.8747) centre (-15.3792, -10.8078) ccw projected
  arc A385 (-11.5547, -16.9334) -> (-11.2226, -17.1553) centre (0, 0) ccw projected
  arc A386 (-11.4485, -16.4566) -> (-11.5547, -16.9334) centre (-4.0998, -18.3445) ccw projected
  arc A387 (-11.3386, -16.0778) -> (-11.4485, -16.4566) centre (-5.2423, -18.051) ccw projected
  arc A388 (-11.2344, -15.7854) -> (-11.3386, -16.0778) centre (-6.3229, -17.7012) ccw projected
  arc A389 (-11.5412, -15.5625) -> (-11.2344, -15.7854) centre (0, 0) ccw projected
  arc A390 (-11.7871, -15.752) -> (-11.5412, -15.5625) centre (-14.881, -11.4834) ccw projected
  arc A391 (-12.1134, -15.9735) -> (-11.7871, -15.752) centre (-15.5476, -10.5638) ccw projected
  arc A392 (-12.534, -16.2219) -> (-12.1134, -15.9735) centre (-16.1798, -9.5679) ccw projected
  arc A393 (-12.8477, -15.9746) -> (-12.534, -16.2219) centre (0, 0) ccw projected
  arc A394 (-12.7043, -15.5076) -> (-12.8477, -15.9746) centre (-5.5264, -17.9663) ccw projected
  arc A395 (-12.5651, -15.1386) -> (-12.7043, -15.5076) centre (-6.6424, -17.5841) ccw projected
  arc A396 (-12.4383, -14.8553) -> (-12.5651, -15.1386) centre (-7.6922, -17.1506) ccw projected
  arc A397 (-12.7266, -14.609) -> (-12.4383, -14.8553) centre (0, 0) ccw projected
  arc A398 (-12.9866, -14.7786) -> (-12.7266, -14.609) centre (-15.7361, -10.2805) ccw projected
  arc A399 (-13.3293, -14.9739) -> (-12.9866, -14.7786) centre (-16.3285, -9.3114) ccw projected
  arc A400 (-13.7681, -15.1885) -> (-13.3293, -14.9739) centre (-16.8806, -8.2689) ccw projected
  arc A401 (-14.0614, -14.9173) -> (-13.7681, -15.1885) centre (0, 0) ccw projected
  arc A402 (-13.8819, -14.463) -> (-14.0614, -14.9173) centre (-6.919, -17.4773) ccw projected
  arc A403 (-13.7141, -14.1061) -> (-13.8819, -14.463) centre (-8.0015, -17.0087) ccw projected
  arc A404 (-13.5655, -13.8336) -> (-13.7141, -14.1061) centre (-9.0141, -16.4942) ccw projected
  arc A405 (-13.8336, -13.5655) -> (-13.5655, -13.8336) centre (0, 0) ccw projected
  arc A406 (-14.1061, -13.7141) -> (-13.8336, -13.5655) centre (-16.4942, -9.0141) ccw projected
  arc A407 (-14.463, -13.8819) -> (-14.1061, -13.7141) centre (-17.0087, -8.0015) ccw projected
  arc A408 (-14.9173, -14.0614) -> (-14.463, -13.8819) centre (-17.4773, -6.919) ccw projected
  arc A409 (-15.1885, -13.7681) -> (-14.9173, -14.0614) centre (0, 0) ccw projected
  arc A410 (-14.9739, -13.3293) -> (-15.1885, -13.7681) centre (-8.2689, -16.8806) ccw projected
  arc A411 (-14.7786, -12.9866) -> (-14.9739, -13.3293) centre (-9.3114, -16.3285) ccw projected
  arc A412 (-14.609, -12.7266) -> (-14.7786, -12.9866) centre (-10.2805, -15.7361) ccw projected
  arc A413 (-14.8553, -12.4383) -> (-14.609, -12.7266) centre (0, 0) ccw projected
  arc A414 (-15.1386, -12.5651) -> (-14.8553, -12.4383) centre (-17.1506, -7.6922) ccw projected
  arc A415 (-15.5076, -12.7043) -> (-15.1386, -12.5651) centre (-17.5841, -6.6424) ccw projected
  arc A416 (-15.9746, -12.8477) -> (-15.5076, -12.7043) centre (-17.9663, -5.5264) ccw projected
  arc A417 (-16.2219, -12.534) -> (-15.9746, -12.8477) centre (0, 0) ccw projected
  arc A418 (-15.9735, -12.1134) -> (-16.2219, -12.534) centre (-9.5679, -16.1798) ccw projected
  arc A419 (-15.752, -11.7871) -> (-15.9735, -12.1134) centre (-10.5638, -15.5476) ccw projected
  arc A420 (-15.5625, -11.5412) -> (-15.752, -11.7871) centre (-11.4834, -14.881) ccw projected
  arc A421 (-15.7854, -11.2344) -> (-15.5625, -11.5412) centre (0, 0) ccw projected
  arc A422 (-16.0778, -11.3386) -> (-15.7854, -11.2344) centre (-17.7012, -6.3229) ccw projected
  arc A423 (-16.4566, -11.4485) -> (-16.0778, -11.3386) centre (-18.051, -5.2423) ccw projected
  arc A424 (-16.9334, -11.5547) -> (-16.4566, -11.4485) centre (-18.3445, -4.0998) ccw projected
  arc A425 (-17.1553, -11.2226) -> (-16.9334, -11.5547) centre (0, 0) ccw projected
  arc A426 (-16.8747, -10.8227) -> (-17.1553, -11.2226) centre (-10.8078, -15.3792) ccw projected
  arc A427 (-16.6282, -10.5148) -> (-16.8747, -10.8227) centre (-11.7511, -14.6708) ccw projected
  arc A428 (-16.42, -10.2846) -> (-16.6282, -10.5148) centre (-12.6156, -13.9341) ccw projected
  arc A429 (-16.6182, -9.9612) -> (-16.42, -10.2846) centre (0, 0) ccw projected
  arc A430 (-16.9178, -10.0422) -> (-16.6182, -9.9612) centre (-18.1428, -4.9146) ccw projected
  arc A431 (-17.3041, -10.122) -> (-16.9178, -10.0422) centre (-18.4067, -3.8099) ccw projected
  arc A432 (-17.7877, -10.1905) -> (-17.3041, -10.122) centre (-18.6096, -2.6478) ccw projected
  arc A433 (-17.9829, -9.842) -> (-17.7877, -10.1905) centre (0, 0) ccw projected
  arc A434 (-17.6718, -9.4654) -> (-17.9829, -9.842) centre (-11.9812, -14.4838) ccw projected
  arc A435 (-17.4019, -9.1778) -> (-17.6718, -9.4654) centre (-12.8659, -13.7036) ccw projected
  arc A436 (-17.1763, -8.9646) -> (-17.4019, -9.1778) centre (-13.6699, -12.9014) ccw projected
  arc A437 (-17.3485, -8.6267) -> (-17.1763, -8.9646) centre (0, 0) ccw projected
  arc A438 (-17.6536, -8.6839) -> (-17.3485, -8.6267) centre (-18.4724, -3.476) ccw projected
  arc A439 (-18.0449, -8.7331) -> (-17.6536, -8.6839) centre (-18.6488, -2.3539) ccw projected
  arc A440 (-18.5324, -8.7635) -> (-18.0449, -8.7331) centre (-18.76, -1.1796) ccw projected
  arc A441 (-18.6997, -8.4007) -> (-18.5324, -8.7635) centre (0, 0) ccw projected
  arc A442 (-18.36, -8.0497) -> (-18.6997, -8.4007) centre (-13.0806, -13.4991) ccw projected
  arc A443 (-18.0684, -7.7842) -> (-18.36, -8.0497) centre (-13.9014, -12.6519) ccw projected
  arc A444 (-17.8267, -7.5893) -> (-18.0684, -7.7842) centre (-14.64, -11.7891) ccw projected
  arc A445 (-17.9719, -7.2389) -> (-17.8267, -7.5893) centre (0, 0) ccw projected
  arc A446 (-18.2805, -7.272) -> (-17.9719, -7.2389) centre (-18.6882, -2.0159) ccw projected
  arc A447 (-18.6745, -7.2904) -> (-18.2805, -7.272) centre (-18.776, -0.8835) ccw projected
  arc A448 (-19.1629, -7.2825) -> (-18.6745, -7.2904) centre (-18.7947, 0.2959) ccw projected
  arc A449 (-19.3011, -6.9077) -> (-19.1629, -7.2825) centre (0, 0) ccw projected
  arc A450 (-18.9349, -6.5844) -> (-19.3011, -6.9077) centre (-14.0994, -12.4312) ccw projected
  arc A451 (-18.6234, -6.3425) -> (-18.9349, -6.5844) centre (-14.8512, -11.5222) ccw projected
  arc A452 (-18.3672, -6.1673) -> (-18.6234, -6.3425) centre (-15.5199, -10.6041) ccw projected
  arc A453 (-18.4844, -5.8066) -> (-18.3672, -6.1673) centre (0, 0) ccw projected
  arc A454 (-18.7947, -5.8154) -> (-18.4844, -5.8066) centre (-18.7888, -0.5434) ccw projected
  arc A455 (-19.1889, -5.8028) -> (-18.7947, -5.8154) centre (-18.7875, 0.5924) ccw projected
  arc A456 (-19.6752, -5.7565) -> (-19.1889, -5.8028) centre (-18.7136, 1.7696) ccw projected
  arc A457 (-19.7836, -5.372) -> (-19.6752, -5.7565) centre (0, 0) ccw projected
  arc A458 (-19.3932, -5.0785) -> (-19.7836, -5.372) centre (-15.0313, -11.2867) ccw projected
  arc A459 (-19.0636, -4.8618) -> (-19.3932, -5.0785) centre (-15.7095, -10.3215) ccw projected
  arc A460 (-18.7945, -4.7072) -> (-19.0636, -4.8618) centre (-16.304, -9.3537) ccw projected
  arc A461 (-18.883, -4.3384) -> (-18.7945, -4.7072) centre (0, 0) ccw projected
  arc A462 (-19.193, -4.3228) -> (-18.883, -4.3384) centre (-18.7735, 0.9324) ccw projected
  arc A463 (-19.585, -4.2793) -> (-19.193, -4.3228) centre (-18.6831, 2.0646) ccw projected
  arc A464 (-20.0662, -4.1951) -> (-19.585, -4.2793) centre (-18.517, 3.2324) ccw projected
  arc A465 (-20.1441, -3.8033) -> (-20.0662, -4.1951) centre (0, 0) ccw projected
  arc A466 (-19.7318, -3.5413) -> (-20.1441, -3.8033) centre (-15.8705, -10.0726) ccw projected
  arc A467 (-19.3863, -3.3511) -> (-19.7318, -3.5413) centre (-16.4708, -9.0571) ccw projected
  arc A468 (-19.1059, -3.2181) -> (-19.3863, -3.3511) centre (-16.9876, -8.0457) ccw projected
  arc A469 (-19.1652, -2.8435) -> (-19.1059, -3.2181) centre (0, 0) ccw projected
  arc A470 (-19.473, -2.8036) -> (-19.1652, -2.8435) centre (-18.6425, 2.4025) ccw projected
  arc A471 (-19.8604, -2.7295) -> (-19.473, -2.8036) centre (-18.4635, 3.5241) ccw projected
  arc A472 (-20.3335, -2.6078) -> (-19.8604, -2.7295) centre (-18.2064, 4.6753) ccw projected
  arc A473 (-20.3804, -2.2111) -> (-20.3335, -2.6078) centre (0, 0) ccw projected
  arc A474 (-19.9489, -1.9822) -> (-20.3804, -2.2111) centre (-16.6119, -8.7963) ccw projected
  arc A475 (-19.5895, -1.8197) -> (-19.9489, -1.9822) centre (-17.1307, -7.7369) ccw projected
  arc A476 (-19.2995, -1.7091) -> (-19.5895, -1.8197) centre (-17.5665, -6.6881) ccw projected
  arc A477 (-19.3292, -1.331) -> (-19.2995, -1.7091) centre (0, 0) ccw projected
  arc A478 (-19.633, -1.2671) -> (-19.3292, -1.331) centre (-18.3965, 3.8577) ccw projected
  arc A479 (-20.0133, -1.1629) -> (-19.633, -1.2671) centre (-18.1301, 4.9618) ccw projected
  arc A480 (-20.4754, -1.0044) -> (-20.0133, -1.1629) centre (-17.7834, 6.0894) ccw projected
  arc A481 (-20.4911, -0.6052) -> (-20.4754, -1.0044) centre (0, 0) ccw projected
  arc A482 (-20.0429, -0.4109) -> (-20.4911, -0.6052) centre (-17.2508, -7.4658) ccw projected
  arc A483 (-19.6719, -0.2771) -> (-20.0429, -0.4109) centre (-17.6849, -6.369) ccw projected
  arc A484 (-19.3741, -0.1896) -> (-19.6719, -0.2771) centre (-18.0371, -5.2892) ccw projected
  arc A485 (-19.3741, 0.1896) -> (-19.3741, -0.1896) centre (0, 0) ccw projected
  arc A486 (-19.6719, 0.2771) -> (-19.3741, 0.1896) centre (-18.0371, 5.2892) ccw projected
  arc A487 (-20.0429, 0.4109) -> (-19.6719, 0.2771) centre (-17.6849, 6.369) ccw projected
  arc A488 (-20.4911, 0.6052) -> (-20.0429, 0.4109) centre (-17.2508, 7.4658) ccw projected
  arc A489 (-20.4754, 1.0044) -> (-20.4911, 0.6052) centre (0, 0) ccw projected
  arc A490 (-20.0133, 1.1629) -> (-20.4754, 1.0044) centre (-17.7834, -6.0894) ccw projected
  arc A491 (-19.633, 1.2671) -> (-20.0133, 1.1629) centre (-18.1301, -4.9618) ccw projected
  arc A492 (-19.3292, 1.331) -> (-19.633, 1.2671) centre (-18.3965, -3.8577) ccw projected
  arc A493 (-19.2995, 1.7091) -> (-19.3292, 1.331) centre (0, 0) ccw projected
  arc A494 (-19.5895, 1.8197) -> (-19.2995, 1.7091) centre (-17.5665, 6.6881) ccw projected
  arc A495 (-19.9489, 1.9822) -> (-19.5895, 1.8197) centre (-17.1307, 7.7369) ccw projected
  arc A496 (-20.3804, 2.2111) -> (-19.9489, 1.9822) centre (-16.6119, 8.7963) ccw projected
  arc A497 (-20.3335, 2.6078) -> (-20.3804, 2.2111) centre (0, 0) ccw projected
  arc A498 (-19.8604, 2.7295) -> (-20.3335, 2.6078) centre (-18.2064, -4.6753) ccw projected
  arc A499 (-19.473, 2.8036) -> (-19.8604, 2.7295) centre (-18.4635, -3.5241) ccw projected
  arc A500 (-19.1652, 2.8435) -> (-19.473, 2.8036) centre (-18.6425, -2.4025) ccw projected
  arc A501 (-19.1059, 3.2181) -> (-19.1652, 2.8435) centre (0, 0) ccw projected
  arc A502 (-19.3863, 3.3511) -> (-19.1059, 3.2181) centre (-16.9876, 8.0457) ccw projected
  arc A503 (-19.7318, 3.5413) -> (-19.3863, 3.3511) centre (-16.4708, 9.0571) ccw projected
  arc A504 (-20.1441, 3.8033) -> (-19.7318, 3.5413) centre (-15.8705, 10.0726) ccw projected
  arc A505 (-20.0662, 4.1951) -> (-20.1441, 3.8033) centre (0, 0) ccw projected
  arc A506 (-19.585, 4.2793) -> (-20.0662, 4.1951) centre (-18.517, -3.2324) ccw projected
  arc A507 (-19.193, 4.3228) -> (-19.585, 4.2793) centre (-18.6831, -2.0646) ccw projected
  arc A508 (-18.883, 4.3384) -> (-19.193, 4.3228) centre (-18.7735, -0.9324) ccw projected
  arc A509 (-18.7945, 4.7072) -> (-18.883, 4.3384) centre (0, 0) ccw projected
  arc A510 (-19.0636, 4.8618) -> (-18.7945, 4.7072) centre (-16.304, 9.3537) ccw projected
  arc A511 (-19.3932, 5.0785) -> (-19.0636, 4.8618) centre (-15.7095, 10.3215) ccw projected
  arc A512 (-19.7836, 5.372) -> (-19.3932, 5.0785) centre (-15.0313, 11.2867) ccw projected
  arc A513 (-19.6752, 5.7565) -> (-19.7836, 5.372) centre (0, 0) ccw projected
  arc A514 (-19.1889, 5.8028) -> (-19.6752, 5.7565) centre (-18.7136, -1.7696) ccw projected
  arc A515 (-18.7947, 5.8154) -> (-19.1889, 5.8028) centre (-18.7875, -0.5924) ccw projected
  arc A516 (-18.4844, 5.8066) -> (-18.7947, 5.8154) centre (-18.7888, 0.5434) ccw projected
  arc A517 (-18.3672, 6.1673) -> (-18.4844, 5.8066) centre (0, 0) ccw projected
  arc A518 (-18.6234, 6.3425) -> (-18.3672, 6.1673) centre (-15.5199, 10.6041) ccw projected
  arc A519 (-18.9349, 6.5844) -> (-18.6234, 6.3425) centre (-14.8512, 11.5222) ccw projected
  arc A520 (-19.3011, 6.9077) -> (-18.9349, 6.5844) centre (-14.0994, 12.4312) ccw projected
  arc A521 (-19.1629, 7.2825) -> (-19.3011, 6.9077) centre (0, 0) ccw projected
  arc A522 (-18.6745, 7.2904) -> (-19.1629, 7.2825) centre (-18.7947, -0.2959) ccw projected
  arc A523 (-18.2805, 7.272) -> (-18.6745, 7.2904) centre (-18.776, 0.8835) ccw projected
  arc A524 (-17.9719, 7.2389) -> (-18.2805, 7.272) centre (-18.6882, 2.0159) ccw projected
  arc A525 (-17.8267, 7.5893) -> (-17.9719, 7.2389) centre (0, 0) ccw projected
  arc A526 (-18.0684, 7.7842) -> (-17.8267, 7.5893) centre (-14.64, 11.7891) ccw projected
  arc A527 (-18.36, 8.0497) -> (-18.0684, 7.7842) centre (-13.9014, 12.6519) ccw projected
  arc A528 (-18.6997, 8.4007) -> (-18.36, 8.0497) centre (-13.0806, 13.4991) ccw projected
  arc A529 (-18.5324, 8.7635) -> (-18.6997, 8.4007) centre (0, 0) ccw projected
  arc A530 (-18.0449, 8.7331) -> (-18.5324, 8.7635) centre (-18.76, 1.1796) ccw projected
  arc A531 (-17.6536, 8.6839) -> (-18.0449, 8.7331) centre (-18.6488, 2.3539) ccw projected
  arc A532 (-17.3485, 8.6267) -> (-17.6536, 8.6839) centre (-18.4724, 3.476) ccw projected
  arc A533 (-17.1763, 8.9646) -> (-17.3485, 8.6267) centre (0, 0) ccw projected
  arc A534 (-17.4019, 9.1778) -> (-17.1763, 8.9646) centre (-13.6699, 12.9014) ccw projected
  arc A535 (-17.6718, 9.4654) -> (-17.4019, 9.1778) centre (-12.8659, 13.7036) ccw projected
  arc A536 (-17.9829, 9.842) -> (-17.6718, 9.4654) centre (-11.9812, 14.4838) ccw projected
  arc A537 (-17.7877, 10.1905) -> (-17.9829, 9.842) centre (0, 0) ccw projected
  arc A538 (-17.3041, 10.122) -> (-17.7877, 10.1905) centre (-18.6096, 2.6478) ccw projected
  arc A539 (-16.9178, 10.0422) -> (-17.3041, 10.122) centre (-18.4067, 3.8099) ccw projected
  arc A540 (-16.6182, 9.9612) -> (-16.9178, 10.0422) centre (-18.1428, 4.9146) ccw projected
  arc A541 (-16.42, 10.2846) -> (-16.6182, 9.9612) centre (0, 0) ccw projected
  arc A542 (-16.6282, 10.5148) -> (-16.42, 10.2846) centre (-12.6156, 13.9341) ccw projected
  arc A543 (-16.8747, 10.8227) -> (-16.6282, 10.5148) centre (-11.7511, 14.6708) ccw projected
  arc A544 (-17.1553, 11.2226) -> (-16.8747, 10.8227) centre (-10.8078, 15.3792) ccw projected
  arc A545 (-16.9334, 11.5547) -> (-17.1553, 11.2226) centre (0, 0) ccw projected
  arc A546 (-16.4566, 11.4485) -> (-16.9334, 11.5547) centre (-18.3445, 4.0998) ccw projected
  arc A547 (-16.0778, 11.3386) -> (-16.4566, 11.4485) centre (-18.051, 5.2423) ccw projected
  arc A548 (-15.7854, 11.2344) -> (-16.0778, 11.3386) centre (-17.7012, 6.3229) ccw projected
  arc A549 (-15.5625, 11.5412) -> (-15.7854, 11.2344) centre (0, 0) ccw projected
  arc A550 (-15.752, 11.7871) -> (-15.5625, 11.5412) centre (-11.4834, 14.881) ccw projected
  arc A551 (-15.9735, 12.1134) -> (-15.752, 11.7871) centre (-10.5638, 15.5476) ccw projected
  arc A552 (-16.2219, 12.534) -> (-15.9735, 12.1134) centre (-9.5679, 16.1798) ccw projected
  arc A553 (-15.9746, 12.8477) -> (-16.2219, 12.534) centre (0, 0) ccw projected
  arc A554 (-15.5076, 12.7043) -> (-15.9746, 12.8477) centre (-17.9663, 5.5264) ccw projected
  arc A555 (-15.1386, 12.5651) -> (-15.5076, 12.7043) centre (-17.5841, 6.6424) ccw projected
  arc A556 (-14.8553, 12.4383) -> (-15.1386, 12.5651) centre (-17.1506, 7.6922) ccw projected
  arc A557 (-14.609, 12.7266) -> (-14.8553, 12.4383) centre (0, 0) ccw projected
  arc A558 (-14.7786, 12.9866) -> (-14.609, 12.7266) centre (-10.2805, 15.7361) ccw projected
  arc A559 (-14.9739, 13.3293) -> (-14.7786, 12.9866) centre (-9.3114, 16.3285) ccw projected
  arc A560 (-15.1885, 13.7681) -> (-14.9739, 13.3293) centre (-8.2689, 16.8806) ccw projected
  arc A561 (-14.9173, 14.0614) -> (-15.1885, 13.7681) centre (0, 0) ccw projected
  arc A562 (-14.463, 13.8819) -> (-14.9173, 14.0614) centre (-17.4773, 6.919) ccw projected
  arc A563 (-14.1061, 13.7141) -> (-14.463, 13.8819) centre (-17.0087, 8.0015) ccw projected
  arc A564 (-13.8336, 13.5655) -> (-14.1061, 13.7141) centre (-16.4942, 9.0141) ccw projected
  arc A565 (-13.5655, 13.8336) -> (-13.8336, 13.5655) centre (0, 0) ccw projected
  arc A566 (-13.7141, 14.1061) -> (-13.5655, 13.8336) centre (-9.0141, 16.4942) ccw projected
  arc A567 (-13.8819, 14.463) -> (-13.7141, 14.1061) centre (-8.0015, 17.0087) ccw projected